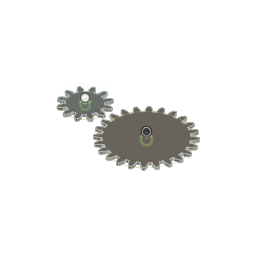
DAY4GEAR.stl (Autodesk Fusion 360 design; units mm, degrees)
part number: 2026-04-16-20-14-41-577
part number: 2026-04-16-20-17-04-548
description: Spur Gear; Module: 12.7; Num Teeth: 12; Pressure Angle: 20.0; Backlash: 0.00 mm
part number: 2026-04-16-20-42-38-505
part number: 2026-04-16-21-00-37-450
part number: 2026-04-16-21-02-31-735
Autodesk Fusion 360 part; units mm, degrees
(part 1 of 5)
sketch "Base Circle" plane through (0, 0, 0) normal (0, 0, 1) x (1, 0, 0) in component "Spur Gear 24 teeth"
  circle A0 centre (0, 0) radius 137.7061
  circle A1 centre (0, 0) radius 5
extrude "Extrude1" add sketch "Base Circle" along normal blind 10 makes body 1 in component "Spur Gear 24 teeth"
sketch "Gear Tooth" plane through (0, 0, 0) normal (0, 0, 1) x (1, 0, 0) in component "Spur Gear 24 teeth"
  spline S0 degree 5 poles (142.7471, -11.4951) (142.8118, -11.5003) (142.9412, -11.5091) (143.1354, -11.5173) (143.3946, -11.5189) (143.7188, -11.5082) (144.0432, -11.4883) (144.3678, -11.4628) (144.6924, -11.4343) (145.0169, -11.4038) (145.3415, -11.3711) (145.666, -11.3355) (145.9905, -11.2961) (146.3148, -11.2522) (146.6391, -11.2039) (146.9633, -11.1516) (147.2873, -11.0957) (147.6112, -11.037) (147.935, -10.9757) (148.2586, -10.9121) (148.5821, -10.846) (148.9053, -10.7774) (149.2285, -10.7062) (149.5514, -10.6322) (149.8741, -10.5555) (150.1966, -10.4762) (150.5189, -10.3945) (150.8411, -10.3105) (151.1629, -10.2242) (151.4846, -10.1358) (151.806, -10.0451) (152.1272, -9.9523) (152.4482, -9.8574) (152.7689, -9.7602) (153.0893, -9.661) (153.4095, -9.5596) (153.7295, -9.4562) (154.0491, -9.3508) (154.3685, -9.2434) (154.6877, -9.1341) (155.0065, -9.0228) (155.325, -8.9096) (155.6433, -8.7946) (155.9613, -8.6776) (156.279, -8.5588) (156.5963, -8.4382) (156.9134, -8.3157) (157.2301, -8.1914) (157.5466, -8.0654) (157.8627, -7.9376) (158.1785, -7.808) (158.494, -7.6767) (158.8091, -7.5437) (159.1239, -7.409) (159.4384, -7.2727) (159.7525, -7.1346) (160.0663, -6.9949) (160.3798, -6.8535) (160.6929, -6.7105) (161.0056, -6.5659) (161.318, -6.4196) (161.63, -6.2718) (161.9417, -6.1224) (162.253, -5.9714) (162.5639, -5.8189) (162.8745, -5.6648) (163.1846, -5.5091) (163.4944, -5.352) (163.8038, -5.1933) (164.1128, -5.0331) (164.4215, -4.8714) (164.6681, -4.7409) (164.8528, -4.6423) (164.9759, -4.5763) (165.0375, -4.5432) knots 0 0 0 0 0 0 0.01428571 0.02857143 0.04285714 0.05714286 0.07142857 0.08571429 0.1 0.11428571 0.12857143 0.14285714 0.15714286 0.17142857 0.18571429 0.2 0.21428571 0.22857143 0.24285714 0.25714286 0.27142857 0.28571429 0.3 0.31428571 0.32857143 0.34285714 0.35714286 0.37142857 0.38571429 0.4 0.41428571 0.42857143 0.44285714 0.45714286 0.47142857 0.48571429 0.5 0.51428571 0.52857143 0.54285714 0.55714286 0.57142857 0.58571429 0.6 0.61428571 0.62857143 0.64285714 0.65714286 0.67142857 0.68571429 0.7 0.71428571 0.72857143 0.74285714 0.75714286 0.77142857 0.78571429 0.8 0.81428571 0.82857143 0.84285714 0.85714286 0.87142857 0.88571429 0.9 0.91428571 0.92857143 0.94285714 0.95714286 0.97142857 0.98571429 1 1 1 1 1 1
  spline S1 degree 5 poles (142.7471, 11.4951) (142.8118, 11.5003) (142.9412, 11.5091) (143.1354, 11.5173) (143.3946, 11.5189) (143.7188, 11.5082) (144.0432, 11.4883) (144.3678, 11.4628) (144.6924, 11.4343) (145.0169, 11.4038) (145.3415, 11.3711) (145.666, 11.3355) (145.9905, 11.2961) (146.3148, 11.2522) (146.6391, 11.2039) (146.9633, 11.1516) (147.2873, 11.0957) (147.6112, 11.037) (147.935, 10.9757) (148.2586, 10.9121) (148.5821, 10.846) (148.9053, 10.7774) (149.2285, 10.7062) (149.5514, 10.6322) (149.8741, 10.5555) (150.1966, 10.4762) (150.5189, 10.3945) (150.8411, 10.3105) (151.1629, 10.2242) (151.4846, 10.1358) (151.806, 10.0451) (152.1272, 9.9523) (152.4482, 9.8574) (152.7689, 9.7602) (153.0893, 9.661) (153.4095, 9.5596) (153.7295, 9.4562) (154.0491, 9.3508) (154.3685, 9.2434) (154.6877, 9.1341) (155.0065, 9.0228) (155.325, 8.9096) (155.6433, 8.7946) (155.9613, 8.6776) (156.279, 8.5588) (156.5963, 8.4382) (156.9134, 8.3157) (157.2301, 8.1914) (157.5466, 8.0654) (157.8627, 7.9376) (158.1785, 7.808) (158.494, 7.6767) (158.8091, 7.5437) (159.1239, 7.409) (159.4384, 7.2727) (159.7525, 7.1346) (160.0663, 6.9949) (160.3798, 6.8535) (160.6929, 6.7105) (161.0056, 6.5659) (161.318, 6.4196) (161.63, 6.2718) (161.9417, 6.1224) (162.253, 5.9714) (162.5639, 5.8189) (162.8745, 5.6648) (163.1846, 5.5091) (163.4944, 5.352) (163.8038, 5.1933) (164.1128, 5.0331) (164.4215, 4.8714) (164.6681, 4.7409) (164.8528, 4.6423) (164.9759, 4.5763) (165.0375, 4.5432) knots 0 0 0 0 0 0 0.01428571 0.02857143 0.04285714 0.05714286 0.07142857 0.08571429 0.1 0.11428571 0.12857143 0.14285714 0.15714286 0.17142857 0.18571429 0.2 0.21428571 0.22857143 0.24285714 0.25714286 0.27142857 0.28571429 0.3 0.31428571 0.32857143 0.34285714 0.35714286 0.37142857 0.38571429 0.4 0.41428571 0.42857143 0.44285714 0.45714286 0.47142857 0.48571429 0.5 0.51428571 0.52857143 0.54285714 0.55714286 0.57142857 0.58571429 0.6 0.61428571 0.62857143 0.64285714 0.65714286 0.67142857 0.68571429 0.7 0.71428571 0.72857143 0.74285714 0.75714286 0.77142857 0.78571429 0.8 0.81428571 0.82857143 0.84285714 0.85714286 0.87142857 0.88571429 0.9 0.91428571 0.92857143 0.94285714 0.95714286 0.97142857 0.98571429 1 1 1 1 1 1
  arc A0 (165.0375, -4.5432) -> (165.0375, 4.5432) centre (0, 0) ccw
  line L0 (137.2518, -11.0526) -> (142.7471, -11.4951)
  line L1 (137.2518, 11.0526) -> (142.7471, 11.4951)
  line L2 (137.2518, -11.0526) -> (137.2518, 11.0526)
  point P0 (144.318, -11.4661)
  point P1 (145.899, -11.3066)
  point P2 (147.486, -11.0593)
  point P3 (149.0774, -10.7392)
  point P4 (150.672, -10.3543)
  point P5 (152.2688, -9.9102)
  point P6 (153.8671, -9.4106)
  point P7 (155.466, -8.8584)
  point P8 (157.065, -8.256)
  point P9 (158.6633, -7.605)
  point P10 (160.2603, -6.9071)
  point P11 (161.8554, -6.1635)
  point P12 (163.448, -5.3752)
  point P13 (144.318, 11.4661)
  point P14 (145.899, 11.3066)
  point P15 (147.486, 11.0593)
  point P16 (149.0774, 10.7392)
  point P17 (150.672, 10.3543)
  point P18 (152.2688, 9.9102)
  point P19 (153.8671, 9.4106)
  point P20 (155.466, 8.8584)
  point P21 (157.065, 8.256)
  point P22 (158.6633, 7.605)
  point P23 (160.2603, 6.9071)
  point P24 (161.8554, 6.1635)
  point P25 (163.448, 5.3752)
extrude "Extrude2" add sketch "Gear Tooth" along normal blind 10 bodies 1 in component "Spur Gear 24 teeth"
fillet "Fillet1" radius 2 2 edges at (137.2618, -11.0534, 5) (137.2618, 11.0534, 5) on bodies 1 in component "Spur Gear 24 teeth"
pattern_circular "C-Pattern1" count 24 over 360 about axis through (0, 0, 0) along (0, 0, 1) of "Extrude2", "Fillet1" in component "Spur Gear 24 teeth"
sketch "Diametrial Pitch Circle" plane through (0, 0, 0) normal (0, 0, 1) x (1, 0, 0) in component "Spur Gear 24 teeth"
  circle A0 centre (0, 0) radius 152.4 construction
move_face "MoveFace1" by (19.6092, -71.5735, 0) 1 faces at (0.1538, -93.0525, 10) on bodies 1 in component "Spur Gear 24 teeth"
sketch "Base Circle (2)" plane through (0, 0, 0) normal (0, 0, 1) x (1, 0, 0) in component "Spur Gear 12 teeth"
  circle A0 centre (0, 0) radius 61.5061
  circle A1 centre (0, 0) radius 5
extrude "Extrude1'" add sketch "Base Circle (2)" along normal blind 10 separate body makes body 2 in component "Spur Gear 12 teeth"
sketch "Gear Tooth (2)" plane through (0, 0, 0) normal (0, 0, 1) x (1, 0, 0) in component "Spur Gear 12 teeth"
  spline S0 degree 5 poles (70.8448, -10.4033) (70.8965, -10.4109) (71.0001, -10.4244) (71.1558, -10.4396) (71.3641, -10.4502) (71.6254, -10.4506) (71.8873, -10.4416) (72.1496, -10.4272) (72.4121, -10.4097) (72.6748, -10.3901) (72.9374, -10.3683) (73.2002, -10.3433) (73.463, -10.3142) (73.726, -10.2804) (73.989, -10.2421) (74.2521, -10.1996) (74.5151, -10.1535) (74.7781, -10.1045) (75.041, -10.0529) (75.3037, -9.9989) (75.5664, -9.9422) (75.8289, -9.8828) (76.0913, -9.8206) (76.3536, -9.7555) (76.6157, -9.6876) (76.8776, -9.6169) (77.1394, -9.5437) (77.4009, -9.4681) (77.6622, -9.3901) (77.9233, -9.3098) (78.1842, -9.2272) (78.4448, -9.1423) (78.7051, -9.055) (78.9652, -8.9654) (79.225, -8.8736) (79.4846, -8.7796) (79.7438, -8.6834) (80.0027, -8.585) (80.2613, -8.4845) (80.5196, -8.382) (80.7775, -8.2774) (81.0352, -8.1707) (81.2924, -8.062) (81.5493, -7.9513) (81.8059, -7.8386) (82.0621, -7.7239) (82.3179, -7.6073) (82.5733, -7.4887) (82.8283, -7.3682) (83.0829, -7.2459) (83.3371, -7.1216) (83.5909, -6.9955) (83.8443, -6.8676) (84.0972, -6.7378) (84.3497, -6.6062) (84.6018, -6.4728) (84.8534, -6.3376) (85.1045, -6.2006) (85.3552, -6.0619) (85.6054, -5.9214) (85.8552, -5.7792) (86.1044, -5.6353) (86.3532, -5.4897) (86.6015, -5.3423) (86.8493, -5.1933) (87.0965, -5.0426) (87.3433, -4.8902) (87.5895, -4.7362) (87.8352, -4.5806) (88.0804, -4.4233) (88.325, -4.2644) (88.5203, -4.136) (88.6665, -4.039) (88.7639, -3.974) (88.8126, -3.9414) knots 0 0 0 0 0 0 0.01428571 0.02857143 0.04285714 0.05714286 0.07142857 0.08571429 0.1 0.11428571 0.12857143 0.14285714 0.15714286 0.17142857 0.18571429 0.2 0.21428571 0.22857143 0.24285714 0.25714286 0.27142857 0.28571429 0.3 0.31428571 0.32857143 0.34285714 0.35714286 0.37142857 0.38571429 0.4 0.41428571 0.42857143 0.44285714 0.45714286 0.47142857 0.48571429 0.5 0.51428571 0.52857143 0.54285714 0.55714286 0.57142857 0.58571429 0.6 0.61428571 0.62857143 0.64285714 0.65714286 0.67142857 0.68571429 0.7 0.71428571 0.72857143 0.74285714 0.75714286 0.77142857 0.78571429 0.8 0.81428571 0.82857143 0.84285714 0.85714286 0.87142857 0.88571429 0.9 0.91428571 0.92857143 0.94285714 0.95714286 0.97142857 0.98571429 1 1 1 1 1 1
  spline S1 degree 5 poles (70.8448, 10.4033) (70.8965, 10.4109) (71.0001, 10.4244) (71.1558, 10.4396) (71.3641, 10.4502) (71.6254, 10.4506) (71.8873, 10.4416) (72.1496, 10.4272) (72.4121, 10.4097) (72.6748, 10.3901) (72.9374, 10.3683) (73.2002, 10.3433) (73.463, 10.3142) (73.726, 10.2804) (73.989, 10.2421) (74.2521, 10.1996) (74.5151, 10.1535) (74.7781, 10.1045) (75.041, 10.0529) (75.3037, 9.9989) (75.5664, 9.9422) (75.8289, 9.8828) (76.0913, 9.8206) (76.3536, 9.7555) (76.6157, 9.6876) (76.8776, 9.6169) (77.1394, 9.5437) (77.4009, 9.4681) (77.6622, 9.3901) (77.9233, 9.3098) (78.1842, 9.2272) (78.4448, 9.1423) (78.7051, 9.055) (78.9652, 8.9654) (79.225, 8.8736) (79.4846, 8.7796) (79.7438, 8.6834) (80.0027, 8.585) (80.2613, 8.4845) (80.5196, 8.382) (80.7775, 8.2774) (81.0352, 8.1707) (81.2924, 8.062) (81.5493, 7.9513) (81.8059, 7.8386) (82.0621, 7.7239) (82.3179, 7.6073) (82.5733, 7.4887) (82.8283, 7.3682) (83.0829, 7.2459) (83.3371, 7.1216) (83.5909, 6.9955) (83.8443, 6.8676) (84.0972, 6.7378) (84.3497, 6.6062) (84.6018, 6.4728) (84.8534, 6.3376) (85.1045, 6.2006) (85.3552, 6.0619) (85.6054, 5.9214) (85.8552, 5.7792) (86.1044, 5.6353) (86.3532, 5.4897) (86.6015, 5.3423) (86.8493, 5.1933) (87.0965, 5.0426) (87.3433, 4.8902) (87.5895, 4.7362) (87.8352, 4.5806) (88.0804, 4.4233) (88.325, 4.2644) (88.5203, 4.136) (88.6665, 4.039) (88.7639, 3.974) (88.8126, 3.9414) knots 0 0 0 0 0 0 0.01428571 0.02857143 0.04285714 0.05714286 0.07142857 0.08571429 0.1 0.11428571 0.12857143 0.14285714 0.15714286 0.17142857 0.18571429 0.2 0.21428571 0.22857143 0.24285714 0.25714286 0.27142857 0.28571429 0.3 0.31428571 0.32857143 0.34285714 0.35714286 0.37142857 0.38571429 0.4 0.41428571 0.42857143 0.44285714 0.45714286 0.47142857 0.48571429 0.5 0.51428571 0.52857143 0.54285714 0.55714286 0.57142857 0.58571429 0.6 0.61428571 0.62857143 0.64285714 0.65714286 0.67142857 0.68571429 0.7 0.71428571 0.72857143 0.74285714 0.75714286 0.77142857 0.78571429 0.8 0.81428571 0.82857143 0.84285714 0.85714286 0.87142857 0.88571429 0.9 0.91428571 0.92857143 0.94285714 0.95714286 0.97142857 0.98571429 1 1 1 1 1 1
  arc A0 (88.8126, -3.9414) -> (88.8126, 3.9414) centre (0, 0) ccw
  line L0 (60.8436, -8.9346) -> (70.8448, -10.4033)
  line L1 (60.8436, 8.9346) -> (70.8448, 10.4033)
  line L2 (60.8436, -8.9346) -> (60.8436, 8.9346)
  point P0 (72.0894, -10.43)
  point P1 (73.3521, -10.3259)
  point P2 (74.626, -10.1325)
  point P3 (75.908, -9.8637)
  point P4 (77.1959, -9.527)
  point P5 (78.488, -9.1273)
  point P6 (79.7828, -8.6681)
  point P7 (81.0789, -8.1518)
  point P8 (82.375, -7.5804)
  point P9 (83.6699, -6.9554)
  point P10 (84.9622, -6.278)
  point P11 (86.2509, -5.5493)
  point P12 (87.5347, -4.7702)
  point P13 (72.0894, 10.43)
  point P14 (73.3521, 10.3259)
  point P15 (74.626, 10.1325)
  point P16 (75.908, 9.8637)
  point P17 (77.1959, 9.527)
  point P18 (78.488, 9.1273)
  point P19 (79.7828, 8.6681)
  point P20 (81.0789, 8.1518)
  point P21 (82.375, 7.5804)
  point P22 (83.6699, 6.9554)
  point P23 (84.9622, 6.278)
  point P24 (86.2509, 5.5493)
  point P25 (87.5347, 4.7702)
extrude "Extrude2'" add sketch "Gear Tooth (2)" along normal blind 10 bodies 2 in component "Spur Gear 12 teeth"
fillet "Fillet1'" radius 2 2 edges at (60.8535, -8.9361, 5) (60.8535, 8.9361, 5) on bodies 2 in component "Spur Gear 12 teeth"
pattern_circular "C-Pattern1'" count 12 over 360 about axis through (0, 0, 0) along (0, 0, 1) of "Extrude2'", "Fillet1'" in component "Spur Gear 12 teeth"
sketch "Diametrial Pitch Circle (2)" plane through (0, 0, 0) normal (0, 0, 1) x (1, 0, 0) in component "Spur Gear 12 teeth"
  circle A0 centre (0, 0) radius 76.2 construction
sketch "Sketch1" plane through (0, 0, 10) normal (0, 0, 1) x (-1, 0, 0)
  arc A0 (-131.6356, 40.4355) -> (-134.2176, 30.7996) centre (0, 0) ccw
  arc A1 (-136.5863, 29.2914) -> (-134.2176, 30.7996) centre (-136.1669, 31.247) ccw
  line L0 (-136.5863, 29.2914) -> (-140.0254, 30.029)
  spline S0 degree 5 poles (-140.0254, 30.029) (-140.0889, 30.0426) (-140.2161, 30.0682) (-140.4076, 30.1017) (-140.6643, 30.1371) (-140.9872, 30.1688) (-141.3114, 30.1914) (-141.6365, 30.2085) (-141.962, 30.2226) (-142.2878, 30.2347) (-142.6139, 30.2447) (-142.9402, 30.2518) (-143.267, 30.255) (-143.5944, 30.2539) (-143.9222, 30.2483) (-144.2504, 30.2387) (-144.579, 30.2257) (-144.9078, 30.2097) (-145.2368, 30.1912) (-145.5659, 30.1703) (-145.8952, 30.1471) (-146.2247, 30.1213) (-146.5543, 30.0928) (-146.8842, 30.0616) (-147.2141, 30.0277) (-147.5442, 29.9912) (-147.8745, 29.9523) (-148.2048, 29.911) (-148.5352, 29.8675) (-148.8657, 29.8217) (-149.1962, 29.7739) (-149.5267, 29.7238) (-149.8573, 29.6715) (-150.188, 29.6171) (-150.5186, 29.5605) (-150.8493, 29.5018) (-151.18, 29.441) (-151.5107, 29.3782) (-151.8414, 29.3135) (-152.172, 29.2467) (-152.5027, 29.178) (-152.8333, 29.1074) (-153.1638, 29.0349) (-153.4944, 28.9604) (-153.8248, 28.8841) (-154.1552, 28.8059) (-154.4856, 28.7259) (-154.8158, 28.644) (-155.146, 28.5603) (-155.4761, 28.4749) (-155.8061, 28.3877) (-156.136, 28.2987) (-156.4658, 28.208) (-156.7955, 28.1155) (-157.1251, 28.0213) (-157.4546, 27.9254) (-157.7839, 27.8279) (-158.1132, 27.7286) (-158.4422, 27.6277) (-158.7712, 27.5252) (-159.1, 27.4209) (-159.4286, 27.3151) (-159.7571, 27.2077) (-160.0855, 27.0986) (-160.4136, 26.9879) (-160.7417, 26.8757) (-161.0695, 26.7619) (-161.3971, 26.6465) (-161.7246, 26.5296) (-162.0519, 26.4111) (-162.379, 26.2911) (-162.6405, 26.1938) (-162.8366, 26.1202) (-162.9672, 26.0708) (-163.0326, 26.046) knots 0 0 0 0 0 0 0.01428571 0.02857143 0.04285714 0.05714286 0.07142857 0.08571429 0.1 0.11428571 0.12857143 0.14285714 0.15714286 0.17142857 0.18571429 0.2 0.21428571 0.22857143 0.24285714 0.25714286 0.27142857 0.28571429 0.3 0.31428571 0.32857143 0.34285714 0.35714286 0.37142857 0.38571429 0.4 0.41428571 0.42857143 0.44285714 0.45714286 0.47142857 0.48571429 0.5 0.51428571 0.52857143 0.54285714 0.55714286 0.57142857 0.58571429 0.6 0.61428571 0.62857143 0.64285714 0.65714286 0.67142857 0.68571429 0.7 0.71428571 0.72857143 0.74285714 0.75714286 0.77142857 0.78571429 0.8 0.81428571 0.82857143 0.84285714 0.85714286 0.87142857 0.88571429 0.9 0.91428571 0.92857143 0.94285714 0.95714286 0.97142857 0.98571429 1 1 1 1 1 1
  arc A2 (-163.0326, 26.046) -> (-164.2186, 17.0374) centre (0, 0) ccw
  spline S1 degree 5 poles (-164.2186, 17.0374) (-164.1619, 16.9966) (-164.0484, 16.915) (-163.8781, 16.7932) (-163.6507, 16.6316) (-163.3658, 16.431) (-163.0803, 16.2318) (-162.7943, 16.0341) (-162.5077, 15.8379) (-162.2205, 15.6431) (-161.9327, 15.4498) (-161.6443, 15.2579) (-161.3554, 15.0676) (-161.0659, 14.8788) (-160.7758, 14.6915) (-160.4852, 14.5057) (-160.194, 14.3215) (-159.9023, 14.1389) (-159.61, 13.9578) (-159.3171, 13.7783) (-159.0237, 13.6005) (-158.7297, 13.4242) (-158.4351, 13.2495) (-158.1401, 13.0765) (-157.8444, 12.9052) (-157.5482, 12.7355) (-157.2515, 12.5676) (-156.9542, 12.4013) (-156.6564, 12.2368) (-156.358, 12.0739) (-156.0591, 11.9129) (-155.7597, 11.7536) (-155.4597, 11.5962) (-155.1592, 11.4406) (-154.8581, 11.2868) (-154.5565, 11.1349) (-154.2544, 10.9848) (-153.9518, 10.8367) (-153.6486, 10.6904) (-153.3449, 10.5461) (-153.0407, 10.4039) (-152.7359, 10.2636) (-152.4306, 10.1254) (-152.1248, 9.9894) (-151.8185, 9.8555) (-151.5116, 9.7237) (-151.2043, 9.594) (-150.8964, 9.4664) (-150.588, 9.3411) (-150.2791, 9.218) (-149.9697, 9.0973) (-149.6597, 8.9791) (-149.3492, 8.8636) (-149.0382, 8.7508) (-148.7266, 8.6406) (-148.4145, 8.5329) (-148.102, 8.4276) (-147.789, 8.3246) (-147.4755, 8.224) (-147.1615, 8.1264) (-146.847, 8.0321) (-146.5318, 7.9419) (-146.2159, 7.8561) (-145.8994, 7.7747) (-145.5823, 7.6971) (-145.2648, 7.6223) (-144.947, 7.5497) (-144.6289, 7.479) (-144.3105, 7.4114) (-143.9914, 7.3493) (-143.6714, 7.2964) (-143.4142, 7.2641) (-143.2205, 7.247) (-143.0911, 7.2388) (-143.0263, 7.2355) knots -1 -1 -1 -1 -1 -1 -0.98571429 -0.97142857 -0.95714286 -0.94285714 -0.92857143 -0.91428571 -0.9 -0.88571429 -0.87142857 -0.85714286 -0.84285714 -0.82857143 -0.81428571 -0.8 -0.78571429 -0.77142857 -0.75714286 -0.74285714 -0.72857143 -0.71428571 -0.7 -0.68571429 -0.67142857 -0.65714286 -0.64285714 -0.62857143 -0.61428571 -0.6 -0.58571429 -0.57142857 -0.55714286 -0.54285714 -0.52857143 -0.51428571 -0.5 -0.48571429 -0.47142857 -0.45714286 -0.44285714 -0.42857143 -0.41428571 -0.4 -0.38571429 -0.37142857 -0.35714286 -0.34285714 -0.32857143 -0.31428571 -0.3 -0.28571429 -0.27142857 -0.25714286 -0.24285714 -0.22857143 -0.21428571 -0.2 -0.18571429 -0.17142857 -0.15714286 -0.14285714 -0.12857143 -0.11428571 -0.1 -0.08571429 -0.07142857 -0.05714286 -0.04285714 -0.02857143 -0.01428571 0 0 0 0 0 0
  line L1 (-143.0263, 7.2355) -> (-139.5134, 7.0578)
  arc A3 (-137.6157, 4.9879) -> (-139.5134, 7.0578) centre (-139.6144, 5.0603) ccw
  arc A4 (-137.6157, 4.9879) -> (-137.6157, -4.9879) centre (0, 0) ccw
  arc A5 (-139.5134, -7.0578) -> (-137.6157, -4.9879) centre (-139.6144, -5.0603) ccw
  line L2 (-139.5134, -7.0578) -> (-143.0263, -7.2355)
  spline S2 degree 5 poles (-143.0263, -7.2355) (-143.0911, -7.2388) (-143.2205, -7.247) (-143.4142, -7.2641) (-143.6714, -7.2964) (-143.9914, -7.3493) (-144.3105, -7.4114) (-144.6289, -7.479) (-144.947, -7.5497) (-145.2648, -7.6223) (-145.5823, -7.6971) (-145.8994, -7.7747) (-146.2159, -7.8561) (-146.5318, -7.9419) (-146.847, -8.0321) (-147.1615, -8.1264) (-147.4755, -8.224) (-147.789, -8.3246) (-148.102, -8.4276) (-148.4145, -8.5329) (-148.7266, -8.6406) (-149.0382, -8.7508) (-149.3492, -8.8636) (-149.6597, -8.9791) (-149.9697, -9.0973) (-150.2791, -9.218) (-150.588, -9.3411) (-150.8964, -9.4664) (-151.2043, -9.594) (-151.5116, -9.7237) (-151.8185, -9.8555) (-152.1248, -9.9894) (-152.4306, -10.1254) (-152.7359, -10.2636) (-153.0407, -10.4039) (-153.3449, -10.5461) (-153.6486, -10.6904) (-153.9518, -10.8367) (-154.2544, -10.9848) (-154.5565, -11.1349) (-154.8581, -11.2868) (-155.1592, -11.4406) (-155.4597, -11.5962) (-155.7597, -11.7536) (-156.0591, -11.9129) (-156.358, -12.0739) (-156.6564, -12.2368) (-156.9542, -12.4013) (-157.2515, -12.5676) (-157.5482, -12.7355) (-157.8444, -12.9052) (-158.1401, -13.0765) (-158.4351, -13.2495) (-158.7297, -13.4242) (-159.0237, -13.6005) (-159.3171, -13.7783) (-159.61, -13.9578) (-159.9023, -14.1389) (-160.194, -14.3215) (-160.4852, -14.5057) (-160.7758, -14.6915) (-161.0659, -14.8788) (-161.3554, -15.0676) (-161.6443, -15.2579) (-161.9327, -15.4498) (-162.2205, -15.6431) (-162.5077, -15.8379) (-162.7943, -16.0341) (-163.0803, -16.2318) (-163.3658, -16.431) (-163.6507, -16.6316) (-163.8781, -16.7932) (-164.0484, -16.915) (-164.1619, -16.9966) (-164.2186, -17.0374) knots 0 0 0 0 0 0 0.01428571 0.02857143 0.04285714 0.05714286 0.07142857 0.08571429 0.1 0.11428571 0.12857143 0.14285714 0.15714286 0.17142857 0.18571429 0.2 0.21428571 0.22857143 0.24285714 0.25714286 0.27142857 0.28571429 0.3 0.31428571 0.32857143 0.34285714 0.35714286 0.37142857 0.38571429 0.4 0.41428571 0.42857143 0.44285714 0.45714286 0.47142857 0.48571429 0.5 0.51428571 0.52857143 0.54285714 0.55714286 0.57142857 0.58571429 0.6 0.61428571 0.62857143 0.64285714 0.65714286 0.67142857 0.68571429 0.7 0.71428571 0.72857143 0.74285714 0.75714286 0.77142857 0.78571429 0.8 0.81428571 0.82857143 0.84285714 0.85714286 0.87142857 0.88571429 0.9 0.91428571 0.92857143 0.94285714 0.95714286 0.97142857 0.98571429 1 1 1 1 1 1
  arc A6 (-164.2186, -17.0374) -> (-163.0326, -26.046) centre (0, 0) ccw
  spline S3 degree 5 poles (-163.0326, -26.046) (-162.9672, -26.0708) (-162.8366, -26.1202) (-162.6405, -26.1938) (-162.379, -26.2911) (-162.0519, -26.4111) (-161.7246, -26.5296) (-161.3971, -26.6465) (-161.0695, -26.7619) (-160.7417, -26.8757) (-160.4136, -26.9879) (-160.0855, -27.0986) (-159.7571, -27.2077) (-159.4286, -27.3151) (-159.1, -27.4209) (-158.7712, -27.5252) (-158.4422, -27.6277) (-158.1132, -27.7286) (-157.7839, -27.8279) (-157.4546, -27.9254) (-157.1251, -28.0213) (-156.7955, -28.1155) (-156.4658, -28.208) (-156.136, -28.2987) (-155.8061, -28.3877) (-155.4761, -28.4749) (-155.146, -28.5603) (-154.8158, -28.644) (-154.4856, -28.7259) (-154.1552, -28.8059) (-153.8248, -28.8841) (-153.4944, -28.9604) (-153.1638, -29.0349) (-152.8333, -29.1074) (-152.5027, -29.178) (-152.172, -29.2467) (-151.8414, -29.3135) (-151.5107, -29.3782) (-151.18, -29.441) (-150.8493, -29.5018) (-150.5186, -29.5605) (-150.188, -29.6171) (-149.8573, -29.6715) (-149.5267, -29.7238) (-149.1962, -29.7739) (-148.8657, -29.8217) (-148.5352, -29.8675) (-148.2048, -29.911) (-147.8745, -29.9523) (-147.5442, -29.9912) (-147.2141, -30.0277) (-146.8842, -30.0616) (-146.5543, -30.0928) (-146.2247, -30.1213) (-145.8952, -30.1471) (-145.5659, -30.1703) (-145.2368, -30.1912) (-144.9078, -30.2097) (-144.579, -30.2257) (-144.2504, -30.2387) (-143.9222, -30.2483) (-143.5944, -30.2539) (-143.267, -30.255) (-142.9402, -30.2518) (-142.6139, -30.2447) (-142.2878, -30.2347) (-141.962, -30.2226) (-141.6365, -30.2085) (-141.3114, -30.1914) (-140.9872, -30.1688) (-140.6643, -30.1371) (-140.4076, -30.1017) (-140.2161, -30.0682) (-140.0889, -30.0426) (-140.0254, -30.029) knots -1 -1 -1 -1 -1 -1 -0.98571429 -0.97142857 -0.95714286 -0.94285714 -0.92857143 -0.91428571 -0.9 -0.88571429 -0.87142857 -0.85714286 -0.84285714 -0.82857143 -0.81428571 -0.8 -0.78571429 -0.77142857 -0.75714286 -0.74285714 -0.72857143 -0.71428571 -0.7 -0.68571429 -0.67142857 -0.65714286 -0.64285714 -0.62857143 -0.61428571 -0.6 -0.58571429 -0.57142857 -0.55714286 -0.54285714 -0.52857143 -0.51428571 -0.5 -0.48571429 -0.47142857 -0.45714286 -0.44285714 -0.42857143 -0.41428571 -0.4 -0.38571429 -0.37142857 -0.35714286 -0.34285714 -0.32857143 -0.31428571 -0.3 -0.28571429 -0.27142857 -0.25714286 -0.24285714 -0.22857143 -0.21428571 -0.2 -0.18571429 -0.17142857 -0.15714286 -0.14285714 -0.12857143 -0.11428571 -0.1 -0.08571429 -0.07142857 -0.05714286 -0.04285714 -0.02857143 -0.01428571 0 0 0 0 0 0
  line L3 (-140.0254, -30.029) -> (-136.5863, -29.2914)
  arc A7 (-134.2176, -30.7996) -> (-136.5863, -29.2914) centre (-136.1669, -31.247) ccw
  arc A8 (-134.2176, -30.7996) -> (-131.6356, -40.4355) centre (0, 0) ccw
  arc A9 (-132.9329, -42.926) -> (-131.6356, -40.4355) centre (-133.5475, -41.0228) ccw
  line L4 (-132.9329, -42.926) -> (-136.2801, -44.0069)
  spline S4 degree 5 poles (-136.2801, -44.0069) (-136.3418, -44.0268) (-136.4648, -44.0682) (-136.6474, -44.135) (-136.8874, -44.2326) (-137.1829, -44.3666) (-137.475, -44.5092) (-137.7651, -44.6569) (-138.054, -44.8074) (-138.3422, -44.9599) (-138.6296, -45.1143) (-138.9158, -45.2713) (-139.2004, -45.4319) (-139.4833, -45.5965) (-139.7644, -45.7653) (-140.0439, -45.9377) (-140.3219, -46.1133) (-140.5987, -46.2915) (-140.8743, -46.472) (-141.149, -46.6547) (-141.4225, -46.8395) (-141.695, -47.0265) (-141.9662, -47.216) (-142.2362, -47.408) (-142.505, -47.6023) (-142.7727, -47.799) (-143.0392, -47.9978) (-143.3046, -48.1987) (-143.569, -48.4016) (-143.8323, -48.6064) (-144.0946, -48.8132) (-144.3558, -49.0218) (-144.616, -49.2324) (-144.8751, -49.4448) (-145.1332, -49.6592) (-145.3902, -49.8754) (-145.6463, -50.0933) (-145.9012, -50.313) (-146.1552, -50.5345) (-146.4082, -50.7576) (-146.6602, -50.9824) (-146.9112, -51.2089) (-147.1612, -51.437) (-147.4102, -51.6667) (-147.6582, -51.8981) (-147.9053, -52.131) (-148.1513, -52.3655) (-148.3964, -52.6015) (-148.6405, -52.839) (-148.8837, -53.0781) (-149.1259, -53.3186) (-149.3671, -53.5606) (-149.6074, -53.8041) (-149.8467, -54.049) (-150.085, -54.2954) (-150.3224, -54.5432) (-150.5588, -54.7923) (-150.7943, -55.0429) (-151.0289, -55.2948) (-151.2625, -55.5481) (-151.4951, -55.8028) (-151.7268, -56.0587) (-151.9576, -56.316) (-152.1874, -56.5747) (-152.4163, -56.8346) (-152.6442, -57.0958) (-152.8712, -57.3583) (-153.0973, -57.622) (-153.3224, -57.887) (-153.5466, -58.1533) (-153.7698, -58.4208) (-153.9477, -58.6357) (-154.0807, -58.7975) (-154.1692, -58.9056) (-154.2133, -58.9598) knots 0 0 0 0 0 0 0.01428571 0.02857143 0.04285714 0.05714286 0.07142857 0.08571429 0.1 0.11428571 0.12857143 0.14285714 0.15714286 0.17142857 0.18571429 0.2 0.21428571 0.22857143 0.24285714 0.25714286 0.27142857 0.28571429 0.3 0.31428571 0.32857143 0.34285714 0.35714286 0.37142857 0.38571429 0.4 0.41428571 0.42857143 0.44285714 0.45714286 0.47142857 0.48571429 0.5 0.51428571 0.52857143 0.54285714 0.55714286 0.57142857 0.58571429 0.6 0.61428571 0.62857143 0.64285714 0.65714286 0.67142857 0.68571429 0.7 0.71428571 0.72857143 0.74285714 0.75714286 0.77142857 0.78571429 0.8 0.81428571 0.82857143 0.84285714 0.85714286 0.87142857 0.88571429 0.9 0.91428571 0.92857143 0.94285714 0.95714286 0.97142857 0.98571429 1 1 1 1 1 1
  arc A10 (-154.2133, -58.9598) -> (-150.7362, -67.3545) centre (0, 0) ccw
  spline S5 degree 5 poles (-150.7362, -67.3545) (-150.6666, -67.3615) (-150.5276, -67.3754) (-150.3192, -67.3957) (-150.0414, -67.422) (-149.6944, -67.4533) (-149.3476, -67.483) (-149.001, -67.5112) (-148.6547, -67.5378) (-148.3086, -67.5629) (-147.9627, -67.5865) (-147.6171, -67.6084) (-147.2717, -67.6288) (-146.9266, -67.6475) (-146.5817, -67.6647) (-146.2371, -67.6803) (-145.8929, -67.6942) (-145.5489, -67.7065) (-145.2052, -67.7171) (-144.8618, -67.7262) (-144.5188, -67.7335) (-144.176, -67.7392) (-143.8336, -67.7431) (-143.4916, -67.7454) (-143.1499, -67.746) (-142.8085, -67.7448) (-142.4676, -67.7419) (-142.127, -67.7373) (-141.7868, -67.7309) (-141.447, -67.7227) (-141.1076, -67.7127) (-140.7687, -67.7009) (-140.4301, -67.6872) (-140.0921, -67.6718) (-139.7544, -67.6544) (-139.4173, -67.6352) (-139.0806, -67.6141) (-138.7445, -67.5911) (-138.4088, -67.5661) (-138.0736, -67.5392) (-137.739, -67.5103) (-137.405, -67.4794) (-137.0715, -67.4464) (-136.7386, -67.4113) (-136.4064, -67.3741) (-136.0747, -67.3349) (-135.7437, -67.2935) (-135.4133, -67.25) (-135.0836, -67.2044) (-134.7545, -67.1565) (-134.4262, -67.1064) (-134.0987, -67.0537) (-133.772, -66.9985) (-133.4463, -66.9407) (-133.1213, -66.8803) (-132.7972, -66.8175) (-132.4739, -66.7525) (-132.1513, -66.6852) (-131.8296, -66.6155) (-131.5088, -66.5431) (-131.1893, -66.4674) (-130.8712, -66.388) (-130.5548, -66.3044) (-130.2399, -66.2166) (-129.9265, -66.1253) (-129.6142, -66.0313) (-129.3026, -65.9353) (-128.9918, -65.8374) (-128.6822, -65.7368) (-128.3749, -65.631) (-128.0712, -65.5168) (-127.8324, -65.4162) (-127.6561, -65.3342) (-127.5399, -65.2766) (-127.4821, -65.247) knots -1 -1 -1 -1 -1 -1 -0.98571429 -0.97142857 -0.95714286 -0.94285714 -0.92857143 -0.91428571 -0.9 -0.88571429 -0.87142857 -0.85714286 -0.84285714 -0.82857143 -0.81428571 -0.8 -0.78571429 -0.77142857 -0.75714286 -0.74285714 -0.72857143 -0.71428571 -0.7 -0.68571429 -0.67142857 -0.65714286 -0.64285714 -0.62857143 -0.61428571 -0.6 -0.58571429 -0.57142857 -0.55714286 -0.54285714 -0.52857143 -0.51428571 -0.5 -0.48571429 -0.47142857 -0.45714286 -0.44285714 -0.42857143 -0.41428571 -0.4 -0.38571429 -0.37142857 -0.35714286 -0.34285714 -0.32857143 -0.31428571 -0.3 -0.28571429 -0.27142857 -0.25714286 -0.24285714 -0.22857143 -0.21428571 -0.2 -0.18571429 -0.17142857 -0.15714286 -0.14285714 -0.12857143 -0.11428571 -0.1 -0.08571429 -0.07142857 -0.05714286 -0.04285714 -0.02857143 -0.01428571 0 0 0 0 0 0
  line L5 (-127.4821, -65.247) -> (-124.351, -63.6445)
  arc A11 (-121.6727, -64.4882) -> (-124.351, -63.6445) centre (-123.4398, -65.4248) ccw
  arc A12 (-121.6727, -64.4882) -> (-116.6848, -73.1275) centre (0, 0) ccw
  arc A13 (-117.2932, -75.8689) -> (-116.6848, -73.1275) centre (-118.3795, -74.1896) ccw
  line L6 (-117.2932, -75.8689) -> (-120.2466, -77.7792)
  spline S6 degree 5 poles (-120.2466, -77.7792) (-120.3011, -77.8145) (-120.4091, -77.8863) (-120.5683, -77.998) (-120.7749, -78.1545) (-121.0256, -78.3604) (-121.2708, -78.5737) (-121.5128, -78.7915) (-121.7529, -79.0117) (-121.9919, -79.2335) (-122.2295, -79.457) (-122.4652, -79.6828) (-122.6986, -79.9116) (-122.9293, -80.1438) (-123.1571, -80.3795) (-123.3824, -80.6184) (-123.6055, -80.86) (-123.8267, -81.1038) (-124.0463, -81.3495) (-124.2643, -81.597) (-124.4807, -81.8463) (-124.6954, -82.0975) (-124.9084, -82.3507) (-125.1196, -82.606) (-125.3289, -82.8633) (-125.5365, -83.1225) (-125.7425, -83.3836) (-125.9469, -83.6464) (-126.1497, -83.9108) (-126.3511, -84.1768) (-126.5509, -84.4443) (-126.7492, -84.7135) (-126.9461, -84.9842) (-127.1414, -85.2565) (-127.3352, -85.5303) (-127.5275, -85.8057) (-127.7184, -86.0825) (-127.9078, -86.3607) (-128.0958, -86.6403) (-128.2824, -86.9213) (-128.4677, -87.2037) (-128.6515, -87.4874) (-128.8339, -87.7724) (-129.015, -88.0588) (-129.1947, -88.3464) (-129.373, -88.6354) (-129.55, -88.9255) (-129.7257, -89.2169) (-129.9, -89.5096) (-130.073, -89.8034) (-130.2447, -90.0984) (-130.415, -90.3946) (-130.5841, -90.692) (-130.7518, -90.9905) (-130.9183, -91.2902) (-131.0835, -91.5909) (-131.2474, -91.8928) (-131.41, -92.1958) (-131.5713, -92.4998) (-131.7314, -92.805) (-131.8902, -93.1111) (-132.0478, -93.4184) (-132.2041, -93.7266) (-132.3591, -94.0359) (-132.5129, -94.3462) (-132.6655, -94.6575) (-132.8168, -94.9698) (-132.9669, -95.2831) (-133.1158, -95.5973) (-133.2634, -95.9125) (-133.4099, -96.2287) (-133.526, -96.4824) (-133.6126, -96.6731) (-133.6701, -96.8004) (-133.6987, -96.8641) knots 0 0 0 0 0 0 0.01428571 0.02857143 0.04285714 0.05714286 0.07142857 0.08571429 0.1 0.11428571 0.12857143 0.14285714 0.15714286 0.17142857 0.18571429 0.2 0.21428571 0.22857143 0.24285714 0.25714286 0.27142857 0.28571429 0.3 0.31428571 0.32857143 0.34285714 0.35714286 0.37142857 0.38571429 0.4 0.41428571 0.42857143 0.44285714 0.45714286 0.47142857 0.48571429 0.5 0.51428571 0.52857143 0.54285714 0.55714286 0.57142857 0.58571429 0.6 0.61428571 0.62857143 0.64285714 0.65714286 0.67142857 0.68571429 0.7 0.71428571 0.72857143 0.74285714 0.75714286 0.77142857 0.78571429 0.8 0.81428571 0.82857143 0.84285714 0.85714286 0.87142857 0.88571429 0.9 0.91428571 0.92857143 0.94285714 0.95714286 0.97142857 0.98571429 1 1 1 1 1 1
  arc A14 (-133.6987, -96.8641) -> (-128.1673, -104.0728) centre (0, 0) ccw
  spline S7 degree 5 poles (-128.1673, -104.0728) (-128.0984, -104.0616) (-127.9605, -104.039) (-127.7539, -104.0048) (-127.4788, -103.9582) (-127.1355, -103.8986) (-126.7928, -103.8376) (-126.4508, -103.7751) (-126.1093, -103.7112) (-125.7685, -103.6459) (-125.4283, -103.5791) (-125.0888, -103.5108) (-124.7499, -103.4411) (-124.4117, -103.3699) (-124.0741, -103.2972) (-123.7373, -103.2231) (-123.4011, -103.1474) (-123.0657, -103.0703) (-122.731, -102.9916) (-122.397, -102.9114) (-122.0637, -102.8297) (-121.7312, -102.7465) (-121.3994, -102.6617) (-121.0684, -102.5754) (-120.7382, -102.4875) (-120.4088, -102.398) (-120.0802, -102.307) (-119.7524, -102.2143) (-119.4255, -102.1201) (-119.0994, -102.0242) (-118.7742, -101.9268) (-118.4498, -101.8276) (-118.1263, -101.7269) (-117.8038, -101.6244) (-117.4822, -101.5203) (-117.1615, -101.4144) (-116.8418, -101.3069) (-116.523, -101.1977) (-116.2052, -101.0867) (-115.8885, -100.974) (-115.5727, -100.8594) (-115.2581, -100.7431) (-114.9445, -100.6249) (-114.6321, -100.5049) (-114.3207, -100.383) (-114.0106, -100.2592) (-113.7015, -100.1336) (-113.3936, -100.0061) (-113.0869, -99.8767) (-112.7815, -99.7453) (-112.4773, -99.6118) (-112.1746, -99.4762) (-111.8734, -99.3383) (-111.5737, -99.1982) (-111.2754, -99.0558) (-110.9786, -98.9112) (-110.6831, -98.7647) (-110.389, -98.6162) (-110.0962, -98.4657) (-109.8051, -98.3127) (-109.5161, -98.1569) (-109.2294, -97.9978) (-108.9454, -97.8352) (-108.664, -97.6689) (-108.3849, -97.4996) (-108.1075, -97.328) (-107.8314, -97.1546) (-107.5565, -96.9796) (-107.2836, -96.8023) (-107.0141, -96.6205) (-106.7503, -96.4317) (-106.5457, -96.2726) (-106.3966, -96.1478) (-106.2993, -96.0621) (-106.2511, -96.0186) knots -1 -1 -1 -1 -1 -1 -0.98571429 -0.97142857 -0.95714286 -0.94285714 -0.92857143 -0.91428571 -0.9 -0.88571429 -0.87142857 -0.85714286 -0.84285714 -0.82857143 -0.81428571 -0.8 -0.78571429 -0.77142857 -0.75714286 -0.74285714 -0.72857143 -0.71428571 -0.7 -0.68571429 -0.67142857 -0.65714286 -0.64285714 -0.62857143 -0.61428571 -0.6 -0.58571429 -0.57142857 -0.55714286 -0.54285714 -0.52857143 -0.51428571 -0.5 -0.48571429 -0.47142857 -0.45714286 -0.44285714 -0.42857143 -0.41428571 -0.4 -0.38571429 -0.37142857 -0.35714286 -0.34285714 -0.32857143 -0.31428571 -0.3 -0.28571429 -0.27142857 -0.25714286 -0.24285714 -0.22857143 -0.21428571 -0.2 -0.18571429 -0.17142857 -0.15714286 -0.14285714 -0.12857143 -0.11428571 -0.1 -0.08571429 -0.07142857 -0.05714286 -0.04285714 -0.02857143 -0.01428571 0 0 0 0 0 0
  line L7 (-106.2511, -96.0186) -> (-103.6415, -93.6603)
  arc A15 (-100.836, -93.782) -> (-103.6415, -93.6603) centre (-102.3005, -95.1441) ccw
  arc A16 (-100.836, -93.782) -> (-93.782, -100.836) centre (0, 0) ccw
  arc A17 (-93.6603, -103.6415) -> (-93.782, -100.836) centre (-95.1441, -102.3005) ccw
  line L8 (-93.6603, -103.6415) -> (-96.0186, -106.2511)
  spline S8 degree 5 poles (-96.0186, -106.2511) (-96.0621, -106.2993) (-96.1478, -106.3966) (-96.2726, -106.5457) (-96.4317, -106.7503) (-96.6205, -107.0141) (-96.8023, -107.2836) (-96.9796, -107.5565) (-97.1546, -107.8314) (-97.328, -108.1075) (-97.4996, -108.3849) (-97.6689, -108.664) (-97.8352, -108.9454) (-97.9978, -109.2294) (-98.1569, -109.5161) (-98.3127, -109.8051) (-98.4657, -110.0962) (-98.6162, -110.389) (-98.7647, -110.6831) (-98.9112, -110.9786) (-99.0558, -111.2754) (-99.1982, -111.5737) (-99.3383, -111.8734) (-99.4762, -112.1746) (-99.6118, -112.4773) (-99.7453, -112.7815) (-99.8767, -113.0869) (-100.0061, -113.3936) (-100.1336, -113.7015) (-100.2592, -114.0106) (-100.383, -114.3207) (-100.5049, -114.6321) (-100.6249, -114.9445) (-100.7431, -115.2581) (-100.8594, -115.5727) (-100.974, -115.8885) (-101.0867, -116.2052) (-101.1977, -116.523) (-101.3069, -116.8418) (-101.4144, -117.1615) (-101.5203, -117.4822) (-101.6244, -117.8038) (-101.7269, -118.1263) (-101.8276, -118.4498) (-101.9268, -118.7742) (-102.0242, -119.0994) (-102.1201, -119.4255) (-102.2143, -119.7524) (-102.307, -120.0802) (-102.398, -120.4088) (-102.4875, -120.7382) (-102.5754, -121.0684) (-102.6617, -121.3994) (-102.7465, -121.7312) (-102.8297, -122.0637) (-102.9114, -122.397) (-102.9916, -122.731) (-103.0703, -123.0657) (-103.1474, -123.4011) (-103.2231, -123.7373) (-103.2972, -124.0741) (-103.3699, -124.4117) (-103.4411, -124.7499) (-103.5108, -125.0888) (-103.5791, -125.4283) (-103.6459, -125.7685) (-103.7112, -126.1093) (-103.7751, -126.4508) (-103.8376, -126.7928) (-103.8986, -127.1355) (-103.9582, -127.4788) (-104.0048, -127.7539) (-104.039, -127.9605) (-104.0616, -128.0984) (-104.0728, -128.1673) knots 0 0 0 0 0 0 0.01428571 0.02857143 0.04285714 0.05714286 0.07142857 0.08571429 0.1 0.11428571 0.12857143 0.14285714 0.15714286 0.17142857 0.18571429 0.2 0.21428571 0.22857143 0.24285714 0.25714286 0.27142857 0.28571429 0.3 0.31428571 0.32857143 0.34285714 0.35714286 0.37142857 0.38571429 0.4 0.41428571 0.42857143 0.44285714 0.45714286 0.47142857 0.48571429 0.5 0.51428571 0.52857143 0.54285714 0.55714286 0.57142857 0.58571429 0.6 0.61428571 0.62857143 0.64285714 0.65714286 0.67142857 0.68571429 0.7 0.71428571 0.72857143 0.74285714 0.75714286 0.77142857 0.78571429 0.8 0.81428571 0.82857143 0.84285714 0.85714286 0.87142857 0.88571429 0.9 0.91428571 0.92857143 0.94285714 0.95714286 0.97142857 0.98571429 1 1 1 1 1 1
  arc A18 (-104.0728, -128.1673) -> (-96.8641, -133.6987) centre (0, 0) ccw
  spline S9 degree 5 poles (-96.8641, -133.6987) (-96.8004, -133.6701) (-96.6731, -133.6126) (-96.4824, -133.526) (-96.2287, -133.4099) (-95.9125, -133.2634) (-95.5973, -133.1158) (-95.2831, -132.9669) (-94.9698, -132.8168) (-94.6575, -132.6655) (-94.3462, -132.5129) (-94.0359, -132.3591) (-93.7266, -132.2041) (-93.4184, -132.0478) (-93.1111, -131.8902) (-92.805, -131.7314) (-92.4998, -131.5713) (-92.1958, -131.41) (-91.8928, -131.2474) (-91.5909, -131.0835) (-91.2902, -130.9183) (-90.9905, -130.7518) (-90.692, -130.5841) (-90.3946, -130.415) (-90.0984, -130.2447) (-89.8034, -130.073) (-89.5096, -129.9) (-89.2169, -129.7257) (-88.9255, -129.55) (-88.6354, -129.373) (-88.3464, -129.1947) (-88.0588, -129.015) (-87.7724, -128.8339) (-87.4874, -128.6515) (-87.2037, -128.4677) (-86.9213, -128.2824) (-86.6403, -128.0958) (-86.3607, -127.9078) (-86.0825, -127.7184) (-85.8057, -127.5275) (-85.5303, -127.3352) (-85.2565, -127.1414) (-84.9842, -126.9461) (-84.7135, -126.7492) (-84.4443, -126.5509) (-84.1768, -126.3511) (-83.9108, -126.1497) (-83.6464, -125.9469) (-83.3836, -125.7425) (-83.1225, -125.5365) (-82.8633, -125.3289) (-82.606, -125.1196) (-82.3507, -124.9084) (-82.0975, -124.6954) (-81.8463, -124.4807) (-81.597, -124.2643) (-81.3495, -124.0463) (-81.1038, -123.8267) (-80.86, -123.6055) (-80.6184, -123.3824) (-80.3795, -123.1571) (-80.1438, -122.9293) (-79.9116, -122.6986) (-79.6828, -122.4652) (-79.457, -122.2295) (-79.2335, -121.9919) (-79.0117, -121.7529) (-78.7915, -121.5128) (-78.5737, -121.2708) (-78.3604, -121.0256) (-78.1545, -120.7749) (-77.998, -120.5683) (-77.8863, -120.4091) (-77.8145, -120.3011) (-77.7792, -120.2466) knots -1 -1 -1 -1 -1 -1 -0.98571429 -0.97142857 -0.95714286 -0.94285714 -0.92857143 -0.91428571 -0.9 -0.88571429 -0.87142857 -0.85714286 -0.84285714 -0.82857143 -0.81428571 -0.8 -0.78571429 -0.77142857 -0.75714286 -0.74285714 -0.72857143 -0.71428571 -0.7 -0.68571429 -0.67142857 -0.65714286 -0.64285714 -0.62857143 -0.61428571 -0.6 -0.58571429 -0.57142857 -0.55714286 -0.54285714 -0.52857143 -0.51428571 -0.5 -0.48571429 -0.47142857 -0.45714286 -0.44285714 -0.42857143 -0.41428571 -0.4 -0.38571429 -0.37142857 -0.35714286 -0.34285714 -0.32857143 -0.31428571 -0.3 -0.28571429 -0.27142857 -0.25714286 -0.24285714 -0.22857143 -0.21428571 -0.2 -0.18571429 -0.17142857 -0.15714286 -0.14285714 -0.12857143 -0.11428571 -0.1 -0.08571429 -0.07142857 -0.05714286 -0.04285714 -0.02857143 -0.01428571 0 0 0 0 0 0
  line L9 (-77.7792, -120.2466) -> (-75.8689, -117.2932)
  arc A19 (-73.1275, -116.6848) -> (-75.8689, -117.2932) centre (-74.1896, -118.3795) ccw
  arc A20 (-73.1275, -116.6848) -> (-64.4882, -121.6727) centre (0, 0) ccw
  arc A21 (-63.6445, -124.351) -> (-64.4882, -121.6727) centre (-65.4248, -123.4398) ccw
  line L10 (-63.6445, -124.351) -> (-65.247, -127.4821)
  spline S10 degree 5 poles (-65.247, -127.4821) (-65.2766, -127.5399) (-65.3342, -127.6561) (-65.4162, -127.8324) (-65.5168, -128.0712) (-65.631, -128.3749) (-65.7368, -128.6822) (-65.8374, -128.9918) (-65.9353, -129.3026) (-66.0313, -129.6142) (-66.1253, -129.9265) (-66.2166, -130.2399) (-66.3044, -130.5548) (-66.388, -130.8712) (-66.4674, -131.1893) (-66.5431, -131.5088) (-66.6155, -131.8296) (-66.6852, -132.1513) (-66.7525, -132.4739) (-66.8175, -132.7972) (-66.8803, -133.1213) (-66.9407, -133.4463) (-66.9985, -133.772) (-67.0537, -134.0987) (-67.1064, -134.4262) (-67.1565, -134.7545) (-67.2044, -135.0836) (-67.25, -135.4133) (-67.2935, -135.7437) (-67.3349, -136.0747) (-67.3741, -136.4064) (-67.4113, -136.7386) (-67.4464, -137.0715) (-67.4794, -137.405) (-67.5103, -137.739) (-67.5392, -138.0736) (-67.5661, -138.4088) (-67.5911, -138.7445) (-67.6141, -139.0806) (-67.6352, -139.4173) (-67.6544, -139.7544) (-67.6718, -140.0921) (-67.6872, -140.4301) (-67.7009, -140.7687) (-67.7127, -141.1076) (-67.7227, -141.447) (-67.7309, -141.7868) (-67.7373, -142.127) (-67.7419, -142.4676) (-67.7448, -142.8085) (-67.746, -143.1499) (-67.7454, -143.4916) (-67.7431, -143.8336) (-67.7392, -144.176) (-67.7335, -144.5188) (-67.7262, -144.8618) (-67.7171, -145.2052) (-67.7065, -145.5489) (-67.6942, -145.8929) (-67.6803, -146.2371) (-67.6647, -146.5817) (-67.6475, -146.9266) (-67.6288, -147.2717) (-67.6084, -147.6171) (-67.5865, -147.9627) (-67.5629, -148.3086) (-67.5378, -148.6547) (-67.5112, -149.001) (-67.483, -149.3476) (-67.4533, -149.6944) (-67.422, -150.0414) (-67.3957, -150.3192) (-67.3754, -150.5276) (-67.3615, -150.6666) (-67.3545, -150.7362) knots 0 0 0 0 0 0 0.01428571 0.02857143 0.04285714 0.05714286 0.07142857 0.08571429 0.1 0.11428571 0.12857143 0.14285714 0.15714286 0.17142857 0.18571429 0.2 0.21428571 0.22857143 0.24285714 0.25714286 0.27142857 0.28571429 0.3 0.31428571 0.32857143 0.34285714 0.35714286 0.37142857 0.38571429 0.4 0.41428571 0.42857143 0.44285714 0.45714286 0.47142857 0.48571429 0.5 0.51428571 0.52857143 0.54285714 0.55714286 0.57142857 0.58571429 0.6 0.61428571 0.62857143 0.64285714 0.65714286 0.67142857 0.68571429 0.7 0.71428571 0.72857143 0.74285714 0.75714286 0.77142857 0.78571429 0.8 0.81428571 0.82857143 0.84285714 0.85714286 0.87142857 0.88571429 0.9 0.91428571 0.92857143 0.94285714 0.95714286 0.97142857 0.98571429 1 1 1 1 1 1
  arc A22 (-67.3545, -150.7362) -> (-58.9598, -154.2133) centre (0, 0) ccw
  spline S11 degree 5 poles (-58.9598, -154.2133) (-58.9056, -154.1692) (-58.7975, -154.0807) (-58.6357, -153.9477) (-58.4208, -153.7698) (-58.1533, -153.5466) (-57.887, -153.3224) (-57.622, -153.0973) (-57.3583, -152.8712) (-57.0958, -152.6442) (-56.8346, -152.4163) (-56.5747, -152.1874) (-56.316, -151.9576) (-56.0587, -151.7268) (-55.8028, -151.4951) (-55.5481, -151.2625) (-55.2948, -151.0289) (-55.0429, -150.7943) (-54.7923, -150.5588) (-54.5432, -150.3224) (-54.2954, -150.085) (-54.049, -149.8467) (-53.8041, -149.6074) (-53.5606, -149.3671) (-53.3186, -149.1259) (-53.0781, -148.8837) (-52.839, -148.6405) (-52.6015, -148.3964) (-52.3655, -148.1513) (-52.131, -147.9053) (-51.8981, -147.6582) (-51.6667, -147.4102) (-51.437, -147.1612) (-51.2089, -146.9112) (-50.9824, -146.6602) (-50.7576, -146.4082) (-50.5345, -146.1552) (-50.313, -145.9012) (-50.0933, -145.6463) (-49.8754, -145.3902) (-49.6592, -145.1332) (-49.4448, -144.8751) (-49.2324, -144.616) (-49.0218, -144.3558) (-48.8132, -144.0946) (-48.6064, -143.8323) (-48.4016, -143.569) (-48.1987, -143.3046) (-47.9978, -143.0392) (-47.799, -142.7727) (-47.6023, -142.505) (-47.408, -142.2362) (-47.216, -141.9662) (-47.0265, -141.695) (-46.8395, -141.4225) (-46.6547, -141.149) (-46.472, -140.8743) (-46.2915, -140.5987) (-46.1133, -140.3219) (-45.9377, -140.0439) (-45.7653, -139.7644) (-45.5965, -139.4833) (-45.4319, -139.2004) (-45.2713, -138.9158) (-45.1143, -138.6296) (-44.9599, -138.3422) (-44.8074, -138.054) (-44.6569, -137.7651) (-44.5092, -137.475) (-44.3666, -137.1829) (-44.2326, -136.8874) (-44.135, -136.6474) (-44.0682, -136.4648) (-44.0268, -136.3418) (-44.0069, -136.2801) knots -1 -1 -1 -1 -1 -1 -0.98571429 -0.97142857 -0.95714286 -0.94285714 -0.92857143 -0.91428571 -0.9 -0.88571429 -0.87142857 -0.85714286 -0.84285714 -0.82857143 -0.81428571 -0.8 -0.78571429 -0.77142857 -0.75714286 -0.74285714 -0.72857143 -0.71428571 -0.7 -0.68571429 -0.67142857 -0.65714286 -0.64285714 -0.62857143 -0.61428571 -0.6 -0.58571429 -0.57142857 -0.55714286 -0.54285714 -0.52857143 -0.51428571 -0.5 -0.48571429 -0.47142857 -0.45714286 -0.44285714 -0.42857143 -0.41428571 -0.4 -0.38571429 -0.37142857 -0.35714286 -0.34285714 -0.32857143 -0.31428571 -0.3 -0.28571429 -0.27142857 -0.25714286 -0.24285714 -0.22857143 -0.21428571 -0.2 -0.18571429 -0.17142857 -0.15714286 -0.14285714 -0.12857143 -0.11428571 -0.1 -0.08571429 -0.07142857 -0.05714286 -0.04285714 -0.02857143 -0.01428571 0 0 0 0 0 0
  line L11 (-44.0069, -136.2801) -> (-42.926, -132.9329)
  arc A23 (-40.4355, -131.6356) -> (-42.926, -132.9329) centre (-41.0228, -133.5475) ccw
  arc A24 (-40.4355, -131.6356) -> (-30.7996, -134.2176) centre (0, 0) ccw
  arc A25 (-29.2914, -136.5863) -> (-30.7996, -134.2176) centre (-31.247, -136.1669) ccw
  line L12 (-29.2914, -136.5863) -> (-30.029, -140.0254)
  spline S12 degree 5 poles (-30.029, -140.0254) (-30.0426, -140.0889) (-30.0682, -140.2161) (-30.1017, -140.4076) (-30.1371, -140.6643) (-30.1688, -140.9872) (-30.1914, -141.3114) (-30.2085, -141.6365) (-30.2226, -141.962) (-30.2347, -142.2878) (-30.2447, -142.6139) (-30.2518, -142.9402) (-30.255, -143.267) (-30.2539, -143.5944) (-30.2483, -143.9222) (-30.2387, -144.2504) (-30.2257, -144.579) (-30.2097, -144.9078) (-30.1912, -145.2368) (-30.1703, -145.5659) (-30.1471, -145.8952) (-30.1213, -146.2247) (-30.0928, -146.5543) (-30.0616, -146.8842) (-30.0277, -147.2141) (-29.9912, -147.5442) (-29.9523, -147.8745) (-29.911, -148.2048) (-29.8675, -148.5352) (-29.8217, -148.8657) (-29.7739, -149.1962) (-29.7238, -149.5267) (-29.6715, -149.8573) (-29.6171, -150.188) (-29.5605, -150.5186) (-29.5018, -150.8493) (-29.441, -151.18) (-29.3782, -151.5107) (-29.3135, -151.8414) (-29.2467, -152.172) (-29.178, -152.5027) (-29.1074, -152.8333) (-29.0349, -153.1638) (-28.9604, -153.4944) (-28.8841, -153.8248) (-28.8059, -154.1552) (-28.7259, -154.4856) (-28.644, -154.8158) (-28.5603, -155.146) (-28.4749, -155.4761) (-28.3877, -155.8061) (-28.2987, -156.136) (-28.208, -156.4658) (-28.1155, -156.7955) (-28.0213, -157.1251) (-27.9254, -157.4546) (-27.8279, -157.7839) (-27.7286, -158.1132) (-27.6277, -158.4422) (-27.5252, -158.7712) (-27.4209, -159.1) (-27.3151, -159.4286) (-27.2077, -159.7571) (-27.0986, -160.0855) (-26.9879, -160.4136) (-26.8757, -160.7417) (-26.7619, -161.0695) (-26.6465, -161.3971) (-26.5296, -161.7246) (-26.4111, -162.0519) (-26.2911, -162.379) (-26.1938, -162.6405) (-26.1202, -162.8366) (-26.0708, -162.9672) (-26.046, -163.0326) knots 0 0 0 0 0 0 0.01428571 0.02857143 0.04285714 0.05714286 0.07142857 0.08571429 0.1 0.11428571 0.12857143 0.14285714 0.15714286 0.17142857 0.18571429 0.2 0.21428571 0.22857143 0.24285714 0.25714286 0.27142857 0.28571429 0.3 0.31428571 0.32857143 0.34285714 0.35714286 0.37142857 0.38571429 0.4 0.41428571 0.42857143 0.44285714 0.45714286 0.47142857 0.48571429 0.5 0.51428571 0.52857143 0.54285714 0.55714286 0.57142857 0.58571429 0.6 0.61428571 0.62857143 0.64285714 0.65714286 0.67142857 0.68571429 0.7 0.71428571 0.72857143 0.74285714 0.75714286 0.77142857 0.78571429 0.8 0.81428571 0.82857143 0.84285714 0.85714286 0.87142857 0.88571429 0.9 0.91428571 0.92857143 0.94285714 0.95714286 0.97142857 0.98571429 1 1 1 1 1 1
  arc A26 (-26.046, -163.0326) -> (-17.0374, -164.2186) centre (0, 0) ccw